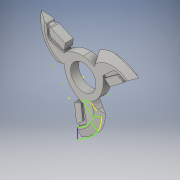
# Autodesk Inventor part: spiner mike
Saved by Autodesk Inventor 2016 (Build 200138000, 138)
## iProperties
Created: 2017-04-28
Part Number: spiner mike
Material: Generic
Document SubType Name: Modeling
Designer: Student
Density: 1 g/cm^3
Appearance: Default
Author: Student
Autodesk Inventor part; units mm, degrees
ref_plane "YZ Plane" through (0, 0, 0) normal (1, 0, 0) x (0, 1, 0)
ref_plane "XZ Plane" through (0, 0, 0) normal (0, 1, 0) x (-1, 0, 0)
ref_plane "XY Plane" through (0, 0, 0) normal (0, 0, 1) x (1, 0, 0)
sketch "Sketch1" plane through (0, 0, 0) normal (0, 0, 1) x (1, 0, 0)
  arc A0 (-8.395, -7.046) -> (9.4916, -5.48) centre (0, 0) ccw
  circle A1 centre (0, 0) radius 10.96
  line L0 (0, 0) -> (0, -50.8) construction
  line L1 (0, 0) -> (43.9941, 25.4) construction
  line L2 (0, 0) -> (-43.9941, 25.4) construction
  line L3 (-4.9194, -48.7335) -> (-4.9194, -39.7784)
  line L4 (-4.9194, -39.7784) -> (-4.4292, -39.0663)
  line L5 (-4.4292, -39.0663) -> (-5.473, -36.6095)
  line L6 (-5.473, -36.6095) -> (-4.4292, -36.6095)
  line L7 (-4.4292, -36.6095) -> (-0.2965, -33.0621)
  line L8 (-0.2965, -33.0621) -> (-1.8424, -20.5791)
  line L9 (-1.8424, -20.5791) -> (-2.7138, -20.2789)
  line L10 (-2.7138, -20.2789) -> (-7.62, -22.3276)
  line L11 (-7.62, -22.3276) -> (-5.9771, -35.5931)
  line L12 (-5.9771, -35.5931) -> (-5.5527, -36.6095)
  line L13 (6.8002, -30.2575) -> (12.771, -34.0606)
  line L14 (12.771, -34.0606) -> (6.8002, -30.2575)
  line L15 (6.8002, -30.2575) -> (8.6862, -24.7835)
  line L16 (8.6862, -24.7835) -> (15.6276, -21.3032)
  arc A2 (-4.9194, -39.7784) -> (6.8002, -30.2575) centre (-15.3955, -14.9095) ccw
  line L17 (-4.4292, -39.0663) -> (1.8493, -34.2708)
  arc A3 (-4.9194, -48.7335) -> (12.771, -34.0606) centre (-26.3902, -4.8468) ccw
  arc A4 (12.771, -34.0606) -> (15.6276, -21.3032) centre (-10.4018, -22.1733) ccw
  arc A5 (15.6276, -21.3032) -> (11.4715, -19.0737) centre (-4.0018, -52.9056) ccw
  line L18 (11.4715, -19.0737) -> (6.2283, -15.2513)
  arc A6 (6.2283, -15.2513) -> (13.7447, -7.9355) centre (-5.413, 4.2285) ccw
  arc A7 (-12.1095, -9.9912) -> (-1.8589, -18.5519) centre (4.7038, -0.2762) ccw
  line L19 (-1.8589, -18.5519) -> (0, -19.6987)
  line L20 (0, -19.6987) -> (2.5904, -31.2604)
  arc A8 (1.8493, -34.2708) -> (2.5904, -31.2604) centre (-2.0693, -31.7097) ccw
  arc A9 (0, -16.8779) -> (8.6862, -24.7835) centre (22.8819, -0.4614) ccw
  line L21 (0, -16.8779) -> (6.2283, -15.2513)
  line L22 (-1.8424, -20.5791) -> (0, -19.6987)
  line L23 (-4.4292, -39.0663) -> (1.8493, -34.2708)
  arc A10 (1.8493, -34.2708) -> (2.5904, -31.2604) centre (-2.8562, -31.516) ccw
  line L24 (2.5904, -31.2604) -> (0, -19.6987)
  line L25 (0, -16.8779) -> (0, -19.6987)
  line L26 (-5.5527, -36.6095) -> (-4.4292, -36.6095)
  arc A11 (-7.6619, -15.2481) -> (0, -16.8779) centre (-0.6585, -1.1487) ccw
  line L27 (9.4916, -5.48) -> (13.7447, -7.9355)
  line L28 (-9.4916, -5.48) -> (-13.2127, -7.6284)
  line L29 (-13.2127, -7.6284) -> (-12.1095, -9.9912)
  line L30 (0, 0) -> (0, 21.6871) construction
  line L31 (0, 0) -> (-30.8731, -17.8246) construction
  line L32 (0, 0) -> (27.4894, -15.871) construction
  point P0 (56.0217, -8.7009)
  dimension "d76" = 10.96
  dimension "d96" = 10.96
  dimension "d133" = 50.8
  dimension "d137" = 360
  dimension "d143" = 48.8574
  dimension "d144" = 26.0439
  dimension "d145" = 48.7335
  dimension "d428" = 120
  dimension "d429" = 120
  constraints: 66 end point, 24 point on circle, 11 centre point, 5 point on line, 4 perpendicular, 3 collinear, 2 vertical, 1 coincident, 1 midpoint, 1 parallel, 14 other
  measures "d96" radius of A0
  measures "d133" distance of L0.start L0.end
  measures "d143" radius of A3
  measures "d144" radius of A4
  measures "d145" vertical distance of point (0, 0) L3.start
  measures "d428" angle of L31 L30
  measures "d429" angle of L32 L30
sketch "Sketch4" plane through (0, 0, 0) normal (0, 0, 1) x (1, 0, 0)
  arc A0 (-4.9194, -48.7335) -> (12.771, -34.0606) centre (-26.3902, -4.8468) ccw projected
  arc A1 (15.6276, -21.3032) -> (11.4715, -19.0737) centre (-4.0018, -52.9056) ccw projected
  line L0 (11.4715, -19.0737) -> (6.2283, -15.2513) projected
  arc A2 (6.2283, -15.2513) -> (12.771, -8.0841) centre (-5.413, 4.2285) ccw projected
  circle A3 centre (0, 0) radius 10.96 projected
  line L1 (-1.8424, -20.5791) -> (0, -19.6987) projected
  line L2 (-1.8424, -20.5791) -> (-2.7138, -20.2789) projected
  line L3 (-2.7138, -20.2789) -> (-7.62, -22.3276) projected
  line L4 (-7.62, -22.3276) -> (-5.9771, -35.5931) projected
  line L5 (-5.9771, -35.5931) -> (-5.5527, -36.6095) projected
  line L6 (-4.4292, -39.0663) -> (-5.473, -36.6095) projected
  line L7 (-4.9194, -39.7784) -> (-4.4292, -39.0663) projected
  line L8 (-4.9194, -48.7335) -> (-4.9194, -39.7784) projected
  arc A4 (-9.4916, -5.48) -> (9.4916, -5.48) centre (0, 0) ccw
  arc A5 (-4.9194, -48.7335) -> (12.771, -34.0606) centre (-26.3902, -4.8468) ccw
  line L9 (15.6276, -21.3032) -> (11.4715, -19.0737)
  line L10 (11.4715, -19.0737) -> (6.2283, -15.2513)
  arc A6 (6.2283, -15.2513) -> (13.7447, -7.9355) centre (-5.413, 4.2285) ccw
  line L11 (13.7447, -7.9355) -> (9.4916, -5.48)
  arc A7 (-9.4916, -5.48) -> (9.4916, -5.48) centre (0, 0) ccw
  line L12 (0, -19.6987) -> (-1.8424, -20.5791)
  line L13 (-1.8424, -20.5791) -> (-2.7138, -20.2789)
  line L14 (-2.7138, -20.2789) -> (-7.62, -22.3276)
  line L15 (-7.62, -22.3276) -> (-5.9771, -35.5931)
  line L16 (-5.5527, -36.6095) -> (-5.9771, -35.5931)
  line L17 (-5.5527, -36.6095) -> (-4.3994, -39.023)
  line L18 (-4.3994, -39.023) -> (-4.9194, -39.7784)
  line L19 (-4.9194, -39.7784) -> (-4.9194, -48.7335)
  line L20 (-4.9194, -39.7784) -> (-4.4292, -39.0663)
  arc A8 (12.771, -34.0606) -> (15.6276, -21.3032) centre (-12.2785, -21.7531) ccw
  line L21 (0, 0) -> (0, 21.3348) construction
  line L22 (0, 0) -> (29.496, -17.0295) construction
  line L23 (0, 0) -> (-39.5645, -22.8426) construction
  line L24 (-9.4916, -5.48) -> (-13.7446, -7.9355)
  arc A9 (-13.7446, -7.9355) -> (0, -19.6987) centre (8.8076, 4.5039) ccw
  dimension "d432" = 120
  dimension "d433" = 120
  dimension "d436" = 4.253
  constraints: 32 end point, 13 point on circle, 6 centre point, 4 collinear, 3 point on line, 2 concentric, 2 vertical, 1 perpendicular, 3 other
  measures "d432" angle of L21 L23
  measures "d433" angle of L21 L22
  measures "d436" horizontal distance of L24.start L24.end
extrude "Extrusion2" add sketch "Sketch4" along normal blind 7 contours L8 L7 L18 L17 L5 L4 L3 L2 L1 A9 L24 A3 L11 A6 L0 L9 A8 A0
sketch "Sketch5" plane through (0, 0, 7) normal (0, 0, 1) x (1, 0, 0)
  line L0 (-1.8424, -20.5791) -> (-2.7138, -20.2789) projected
  line L1 (0, -19.6987) -> (-1.8424, -20.5791) projected
  line L2 (-1.8424, -20.5791) -> (0, -19.6987)
  line L3 (0, -19.6987) -> (2.6364, -31.2668)
  arc A0 (1.9019, -34.2964) -> (2.6364, -31.2668) centre (-1.6228, -31.8381) ccw
  line L4 (-1.8424, -20.5791) -> (-2.7138, -20.2789) projected
  line L5 (-1.8424, -20.5791) -> (-0.3186, -33.0582)
  line L6 (-0.3186, -33.0582) -> (-4.4285, -36.6095)
  line L7 (-5.5527, -36.6095) -> (-4.3994, -39.023) projected
  line L8 (-4.4285, -36.6095) -> (-5.5527, -36.6095)
  line L9 (-5.5527, -36.6095) -> (-4.3994, -39.023)
  line L10 (-4.3994, -39.023) -> (1.9019, -34.2964)
  point P0 (0, 0)
  constraints: 14 end point, 2 collinear, 2 point on circle, 1 centre point, 1 horizontal
extrude "Extrusion3" cut sketch "Sketch5" against normal blind 1.2
sketch "Sketch6" plane through (0, 0, 0) normal (0, 0, -1) x (-1, 0, 0)
  line L0 (0.3186, -33.0582) -> (1.8424, -20.5791) projected
  line L1 (0, -19.6987) -> (-2.6364, -31.2668) projected
  line L2 (1.8424, -20.5791) -> (2.7138, -20.2789) projected
  line L3 (0, -19.6987) -> (1.8424, -20.5791)
  line L4 (1.8424, -20.5791) -> (0, -19.6987) projected
  line L5 (1.8424, -20.5791) -> (0.3186, -33.0582)
  line L6 (0.3186, -33.0582) -> (4.4285, -36.6095)
  line L7 (5.5527, -36.6095) -> (4.4285, -36.6095) projected
  line L8 (4.4285, -36.6095) -> (5.5527, -36.6095)
  line L9 (4.3994, -39.023) -> (4.9194, -39.7784) projected
  line L10 (5.5527, -36.6095) -> (4.3994, -39.023)
  line L11 (4.3994, -39.023) -> (5.5527, -36.6095) projected
  arc A0 (-2.6364, -31.2668) -> (-1.9019, -34.2964) centre (1.6228, -31.8381) ccw projected
  line L12 (4.3994, -39.023) -> (-1.9019, -34.2964)
  arc A1 (-2.6364, -31.2668) -> (-1.9019, -34.2964) centre (1.643, -31.8332) ccw
  line L13 (1.8589, -18.5519) -> (0, -19.6987) projected
  line L14 (-2.6364, -31.2668) -> (0, -19.6987)
  point P0 (0, 0)
  constraints: 14 end point, 3 collinear, 2 point on circle, 1 centre point
extrude "Extrusion4" cut sketch "Sketch6" against normal blind 1.2
sketch "Sketch7" plane through (0, 0, 7) normal (0, 0, 1) x (1, 0, 0)
  line L0 (11.4715, -19.0737) -> (6.2283, -15.2513) projected
  line L1 (6.2283, -15.2513) -> (0, -16.7265)
  arc A0 (0, -16.7265) -> (8.6737, -24.7626) centre (21.5963, -2.1157) ccw
  arc A1 (12.771, -34.0606) -> (15.6276, -21.3032) centre (-12.2785, -21.7531) ccw projected
  line L2 (8.6737, -24.7626) -> (15.6276, -21.3032)
  line L3 (15.6276, -21.3032) -> (8.6737, -24.7626)
  line L4 (8.6737, -24.7626) -> (6.8235, -30.3582)
  line L5 (6.8235, -30.3582) -> (12.771, -34.0606)
  line L6 (12.771, -34.0606) -> (6.8235, -30.3582)
  line L7 (-4.3994, -39.023) -> (-4.9194, -39.7784) projected
  arc A2 (-4.9194, -39.7784) -> (6.8235, -30.3582) centre (-16.7754, -12.97) ccw
  line L8 (-4.9194, -39.7784) -> (-4.9194, -48.6751)
  arc A3 (-4.9194, -48.7335) -> (12.771, -34.0606) centre (-26.3902, -4.8468) ccw projected
  arc A4 (-4.9194, -48.7335) -> (12.771, -34.0606) centre (-26.3902, -4.8468) ccw
  point P0 (0, 0)
  constraints: 14 end point, 6 point on circle, 3 centre point, 2 collinear, 1 vertical
chamfer "Chamfer1" distance 3.5 distance2 7 1 edges at (14.9568, -27.8516, 0) measured on face at (14.9568, -27.8516, 0.5)
chamfer "Chamfer3" distance 7 distance2 3.5 1 edges at (14.9568, -27.8516, 7) measured on face at (14.4688, -27.7423, 7)
pattern_circular "Circular Pattern1" count 3 over 360 about axis through (0, 0, -10) along (0, 0, 1) of "Extrusion4", "Extrusion2", "Extrusion3", "Chamfer1", "Chamfer3"
body "Solid2"
